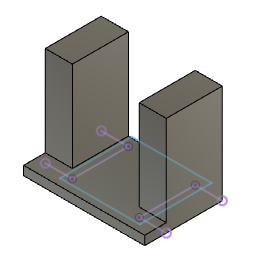
Teatro del mondo v1 (Autodesk Fusion 360 design; units mm, degrees)
Autodesk Fusion 360 part; units mm, degrees
sketch "Sketch1" plane through (0, 0, 0) normal (0, 0, 1) x (1, 0, 0)
  line L0 (0, 0) -> (13400, 0)
  line L1 (13400, 0) -> (13400, 8600)
  line L2 (13400, 8600) -> (0, 8600)
  line L3 (0, 8600) -> (0, 0)
  dimension "d1" = 13400
  dimension "d2" = 8600
  constraint horizontal L0
  constraint vertical L1
  constraint horizontal L2
  constraint vertical L3
  constraint coincident L0.start L3.end
  measures "d1" distance of L0.start L0.end
  measures "d2" distance of L0.start L2.end
extrude "Extrude1" add sketch "Sketch1" along normal blind 1000
sketch "Sketch2" plane through (0, 0, 1000) normal (0, 0, 1) x (-1, 0, 0)
  line L0 (0, -8600) -> (0, 0)
  line L1 (0, 0) -> (-13400, 0)
  line L2 (-13400, 0) -> (-13400, -8600)
  line L3 (-13400, -8600) -> (0, -8600)
  line L4 (0, -8600) -> (-3000, -8600)
  line L5 (-3000, -8600) -> (-3000, -2400)
  line L6 (-3000, -2400) -> (0, -2400)
  line L7 (0, -2400) -> (0, -8600)
  line L8 (-13400, -8600) -> (-10400, -8600)
  line L9 (-10400, -8600) -> (-10400, -2400)
  line L10 (-10400, -2400) -> (-13400, -2400)
  line L11 (-13400, -2400) -> (-13400, -8600)
  constraint horizontal L4
  constraint vertical L5
  constraint horizontal L6
  constraint vertical L7
  constraint coincident L0.start L3.end
  constraint horizontal L8
  constraint vertical L9
  constraint horizontal L10
  constraint vertical L11
  constraint coincident L2.end L3.start
  constraint equal L5 L9
  constraint equal L6 L10
extrude "Extrude2" add sketch "Sketch2" along normal blind 10000 contours L0 L3 L4 L5 L6 L7 | L2 L3 L8 L9 L10 L11
sketch "Sketch3" plane through (0, 0, 0) normal (0, 0, 1) x (1, 0, 0)
  line L0 (2257.1545, 9712.3639) -> (11104.2145, 9712.3639)
  line L1 (11104.2145, 9712.3639) -> (11104.2145, 1780.517)
  line L2 (11104.2145, 1780.517) -> (2257.1545, 1780.517)
  line L3 (2257.1545, 1780.517) -> (2257.1545, 9712.3639)
  line L4 (3000, 2400) -> (3000, 8600)
  line L5 (0, 2400) -> (3000, 2400)
  line L6 (3000, 8600) -> (0, 8600)
  line L7 (13400, 8600) -> (10400, 8600)
  line L8 (10400, 2400) -> (13400, 2400)
  line L9 (10400, 8600) -> (10400, 2400)
  constraint horizontal L0
  constraint vertical L1
  constraint horizontal L2
  constraint vertical L3
